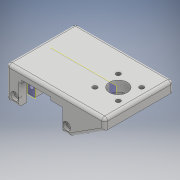
# Autodesk Inventor part: hals
Saved by Autodesk Inventor 2018 (Build 220112000, 112)
## iProperties
Created: 2018-05-22
Part Number: hals
Material: Generic
Document SubType Name: Modeling
Designer: bitbots
Density: 1 g/cm^3
Appearance: Default
Author: bitbots
Autodesk Inventor part; units mm, degrees
ref_plane "YZ Plane" through (0, 0, 0) normal (1, 0, 0) x (0, 1, 0)
ref_plane "XZ Plane" through (0, 0, 0) normal (0, 1, 0) x (-1, 0, 0)
ref_plane "Work Plane1" through (-55.4637, 0, 0.5) normal (0, 0, 1) x (1, 0, 0)
sketch "Sketch1" plane through (-55.4637, 0, 0.5) normal (0, 0, 1) x (1, 0, 0)
  line L0 (-54.3758, 35) -> (-49.4887, 35) projected
  line L1 (-32.4387, 6) -> (-27.5516, 6) projected
  line L2 (-32.4387, 35) -> (-27.5516, 35) projected
  line L3 (-27.5516, 35) -> (-23.5516, 35)
  line L4 (-23.5516, 35) -> (-23.5516, 32.5)
  line L5 (-23.5516, 32.5) -> (-79.5516, 32.5)
  line L6 (-79.5516, 32.5) -> (-79.5516, 8.5)
  line L7 (-79.5516, 8.5) -> (-23.5516, 8.5)
  line L8 (-23.5516, 8.5) -> (-23.5516, 32.5)
  line L9 (-23.5516, 8.5) -> (-22.5516, 8.5)
  line L10 (-22.5516, 8.5) -> (-22.5516, 32.5)
  line L11 (-22.5516, 32.5) -> (-23.5516, 32.5)
  line L12 (-23.5516, 32.5) -> (-23.5516, 8.5)
  point P0 (55.4637, 0)
  dimension "d0" = 4
  dimension "d1" = 2.5
  dimension "d2" = 56
  dimension "d3" = 24
  dimension "d39" = 1
  constraints: 20 end point, 4 parallel, 3 horizontal, 2 perpendicular, 1 vertical
  measures "d0" distance of L2.end L3.end
  measures "d1" distance of L3.end L4.end
  measures "d2" distance of L7.end L6.end
  measures "d3" distance of L6.end L5.end
  measures "d39" distance of L11.end L10.end
extrude "Extrusion1" add sketch "Sketch1" along normal blind 7
ref_plane "Work Plane2" through (-135.0152, 20.5, 7.5) normal (0, 1, 0) x (1, 0, 0)
sketch "Sketch8" plane through (-55.4637, 0, 0.5) normal (0, 0, -1) x (-1, 0, 0)
  circle A0 centre (36.4516, 20.5) radius 5 construction
  circle A1 centre (28.6734, 28.2782) radius 1.025 construction
  circle A2 centre (28.6734, 28.2782) radius 1.5
  circle A3 centre (36.4516, 20.5) radius 6
  circle A4 centre (28.6734, 12.7218) radius 1.5
  circle A5 centre (44.2297, 12.7218) radius 1.5
  circle A6 centre (44.2297, 28.2782) radius 1.5
  point P0 (-55.4637, 0)
  dimension "d40" = 3
  dimension "d41" = 12
  dimension "d44" = 360
  constraints: 5 centre point, 2 coincident, 9 other
  measures "d40" diameter of A2
  measures "d41" diameter of A3
extrude "Extrusion8" cut sketch "Sketch8" against normal through all
sketch "Sketch12" plane through (-55.4637, 0, 0.5) normal (0, 0, -1) x (-1, 0, 0)
  circle A0 centre (44.2297, 28.2782) radius 1.5 construction
  circle A1 centre (28.6734, 12.7218) radius 1.5 construction
  circle A2 centre (28.6734, 28.2782) radius 1.5 construction
  circle A3 centre (44.2297, 12.7218) radius 1.5 construction
  circle A4 centre (36.4516, 20.5) radius 6 construction
  line L0 (79.5516, 8.5) -> (22.5516, 8.5) construction
  line L1 (79.5516, 32.5) -> (79.5516, 8.5) construction
  line L2 (22.5516, 32.5) -> (79.5516, 32.5) construction
  line L3 (22.5516, 8.5) -> (22.5516, 32.5) construction
  circle A5 centre (44.2297, 12.7218) radius 2.75
  circle A6 centre (44.2297, 28.2782) radius 2.75
  circle A7 centre (28.6734, 28.2782) radius 2.75
  circle A8 centre (28.6734, 12.7218) radius 2.75
  point P0 (-55.4637, 0)
  dimension "d66" = 5.5
  dimension "d69" = 360
  constraints: 4 centre point, 1 coincident, 9 other
  measures "d66" diameter of A5
extrude "Extrusion12" cut sketch "Sketch12" against normal blind 3
sketch "Sketch13" plane through (-135.0152, 32.5, 0.5) normal (0, 1, 0) x (1, 0, 0)
  line L0 (57, 0) -> (0, 0) projected
  line L1 (0, 0) -> (0, -7) projected
  line L2 (57, -7) -> (0, -7) projected
  line L3 (57, 0) -> (57, -7) projected
  point P0 (135.0152, 0.5)
extrude "Extrusion13" add sketch "Sketch13" along normal blind 5.5
mirror "Mirror2" about plane through (-135.0152, 20.5, 7.5) normal (0, 1, 0) of "Extrusion13"
sketch "Sketch15" plane through (-135.0152, 38, 0.5) normal (0, 1, 0) x (1, 0, 0)
  line L0 (57, 0) -> (0, 0) construction
  line L1 (0, 0) -> (0, -7) construction
  line L2 (0, -7) -> (57, -7) construction
  line L3 (57, -7) -> (57, 0) construction
  circle A0 centre (-2.819, 9.5) radius 1.35 construction
  circle A1 centre (31.781, 9.5) radius 1.35 construction
  circle A2 centre (-2.819, 9.5) radius 1.5
  circle A3 centre (31.781, 9.5) radius 1.5
  line L4 (0, -3.5) -> (-5, -3.5)
  line L5 (-2.819, 9.5) -> (-2.819, 14.5) construction
  line L6 (-2.819, 9.5) -> (-0.219, 9.5)
  line L7 (-0.219, 9.5) -> (-0.219, 14.5)
  line L8 (-0.219, 14.5) -> (-2.819, 14.5)
  line L9 (-5, -3.5) -> (-5, 14.5)
  line L10 (-5, 14.5) -> (-2.819, 14.5)
  line L11 (31.781, 9.5) -> (29.181, 9.5)
  line L12 (29.181, 9.5) -> (29.181, 14.5)
  line L13 (29.181, 14.5) -> (34.181, 14.5)
  line L14 (-0.219, 9.5) -> (-0.219, -3.5)
  line L15 (29.181, 9.5) -> (29.181, 0)
  line L16 (34.181, 14.5) -> (34.181, 0)
  line L17 (32.5718, 0) -> (38.0718, 0) projected
  line L18 (-5, -3.5) -> (0, -3.5)
  line L19 (0, -3.5) -> (0, -7)
  line L20 (0, -7) -> (-5, -7)
  line L21 (-5, -7) -> (-5, -3.5)
  line L22 (34.181, 0) -> (0, 0)
  line L23 (0, 0) -> (0, -7)
  line L24 (0, -7) -> (34.181, -7)
  line L25 (34.181, -7) -> (34.181, 0)
  line L26 (29.181, 0) -> (34.181, 0)
  line L27 (0, 0) -> (-0.219, 0)
  line L28 (-0.219, 0) -> (-0.219, -3.5)
  line L29 (-0.219, -3.5) -> (0, -3.5)
  line L30 (0, -3.5) -> (0, 0)
  line L31 (34.181, 14.5) -> (57, 0)
  line L32 (57, -7) -> (57, 0) projected
  line L33 (57, 0) -> (57, -7)
  line L34 (36.8218, -7) -> (33.8218, -7) projected
  line L35 (57, -7) -> (33.8218, -7)
  line L36 (34.181, 14.5) -> (34.181, -7)
  line L37 (34.181, -7) -> (57, -7)
  point P0 (135.0152, 0.5)
  dimension "d75" = 3
  dimension "d76" = 3
  dimension "d77" = 5
  dimension "d78" = 5
  dimension "d79" = 2.6
  dimension "d80" = 2.6
  dimension "d81" = 5
  dimension "d82" = 5
  constraints: 62 end point, 10 perpendicular, 8 horizontal, 7 parallel, 4 point on line, 3 collinear, 2 centre point, 2 coincident, 2 vertical, 1 midpoint
  measures "d75" diameter of A2
  measures "d76" diameter of A3
  measures "d77" distance of L4.start L4.end
  measures "d78" distance of L5.start L5.end
  measures "d79" distance of L5.start L6.end
  measures "d80" distance of L11.start L11.end
  measures "d81" distance of L11.end L12.end
  measures "d82" distance of L12.end L13.end
extrude "Extrusion14" add sketch "Sketch15" along normal blind 2
mirror "Mirror3" about plane through (-135.0152, 20.5, 7.5) normal (0, 1, 0) of "Extrusion14"
sketch "Sketch16" plane through (-140.0152, 3, 7.5) normal (0, 1, 0) x (1, 0, 0)
  line L0 (5, 7) -> (5, 0) construction
  line L1 (5, 7) -> (4.781, 7) construction
  line L2 (4.781, 7) -> (4.781, 21.5) construction
  line L3 (4.781, 21.5) -> (0, 21.5) construction
  line L4 (0, 21.5) -> (0, 0) construction
  line L5 (0, 0) -> (5, 0) construction
  circle A0 centre (2.181, 16.5) radius 1.5 construction
  line L6 (0, 21.5) -> (0, 0) construction
  line L7 (0, 0) -> (5, 0) construction
  line L8 (5, 0) -> (4.781, 7) construction
  line L9 (5, 7) -> (5, 0) projected
  line L10 (0, 0) -> (5, 0)
  line L11 (5, 7) -> (4.781, 7) projected
  line L12 (5, 7) -> (4.781, 7)
  line L13 (4.781, 7) -> (0, 11.781)
  line L14 (0, 0) -> (62, 0) projected
  line L15 (0, 11.781) -> (0, 0)
  point P0 (140.0152, 7.5)
  point P1 (39.2, 0)
  dimension "d85" = 135
  constraints: 12 end point, 2 horizontal, 2 perpendicular, 1 point on line
  measures "d85" angle of L12 L13
extrude "Extrusion15" add sketch "Sketch16" along normal up to next
ref_plane "Work Plane3" through (-140.0152, 8.5, -14) normal (0, 1, 0) x (1, 0, 0)
sketch "Sketch17" plane through (-140.0152, 8.5, -14) normal (0, 1, 0) x (1, 0, 0)
  circle A0 centre (2.181, -5) radius 1.5 projected
  circle A1 centre (36.781, -5) radius 1.5 projected
  line L0 (0, -21.5) -> (62, -21.5) construction
  line L1 (62, -21.5) -> (62, -14.5) construction
  line L2 (62, -14.5) -> (39.181, 0) construction
  line L3 (39.181, 0) -> (34.181, 0) construction
  line L4 (34.181, 0) -> (34.181, -14.5) construction
  line L5 (34.181, -14.5) -> (4.781, -14.5) construction
  line L6 (4.781, -14.5) -> (4.781, 0) construction
  line L7 (4.781, 0) -> (0, 0) construction
  line L8 (0, 0) -> (0, -21.5) construction
  line L9 (4.781, -14.5) -> (4.781, 0) projected
  line L10 (0, 0) -> (4.781, 0)
  line L11 (4.781, 0) -> (4.781, -14.5)
  line L12 (4.781, -14.5) -> (0, -14.5)
  line L13 (0, -14.5) -> (0, 0)
  line L14 (41.8218, -21.5) -> (38.8218, -21.5) projected
  line L15 (34.181, 0) -> (40.3218, 0)
  line L16 (40.3218, 0) -> (40.3218, -21.5)
  line L17 (40.3218, -21.5) -> (34.181, -21.5)
  line L18 (34.181, -21.5) -> (34.181, 0)
  point P0 (140.0152, -14)
  constraints: 16 end point, 4 parallel, 2 horizontal, 2 perpendicular, 1 midpoint
extrude "Extrusion16" add sketch "Sketch17" along normal blind 24 contours L12 L13 L10 L9
sketch "Sketch18" plane through (-135.0152, 40, 0.5) normal (0, 1, 0) x (1, 0, 0)
  circle A0 centre (-2.819, 9.5) radius 1.5 projected
  circle A1 centre (31.781, 9.5) radius 1.5 projected
  line L0 (-5, -7) -> (57, -7) projected
  line L1 (57, -7) -> (57, 0) projected
  line L2 (57, 0) -> (34.181, 14.5) projected
  line L3 (34.181, 14.5) -> (29.181, 14.5) projected
  line L4 (29.181, 14.5) -> (29.181, 0) projected
  line L5 (29.181, 0) -> (-0.219, 0) projected
  line L6 (-0.219, 0) -> (-0.219, 14.5) projected
  line L7 (-0.219, 14.5) -> (-5, 14.5) projected
  line L8 (-5, 14.5) -> (-5, -7) projected
  point P0 (135.0152, 0.5)
extrude "Extrusion17" add sketch "Sketch18" along normal blind 1.5
mirror "Mirror4" about plane through (-135.0152, 20.5, 7.5) normal (0, 1, 0) of "Extrusion17"
sketch "Sketch19" plane through (-140.0152, 3, -14) normal (-1, 0, 0) x (0, 0, 1)
  line L0 (6.5, 5.5) -> (6.5, 29.5) projected
  line L1 (9.719, 0) -> (9.719, 5.5) projected
  line L2 (0, 0) -> (9.719, 0) projected
  line L3 (0, 0) -> (0, -3.5) projected
  line L4 (0, -3.5) -> (21.5, -3.5) projected
  line L5 (21.5, -3.5) -> (21.5, 38.5) projected
  line L6 (0, 38.5) -> (21.5, 38.5) projected
  line L7 (0, 35) -> (0, 38.5) projected
  line L8 (0, 35) -> (9.719, 35) projected
  line L9 (9.719, 29.5) -> (9.719, 35) projected
  line L10 (0, 29.5) -> (9.719, 29.5) projected
  line L11 (0, 5.5) -> (0, 29.5) projected
  line L12 (0, 5.5) -> (9.719, 5.5) projected
  point P0 (14, -3)
extrude "Extrusion18" add sketch "Sketch19" along normal blind 1.5
sketch "Sketch20" plane through (-141.5152, 3, -14) normal (-1, 0, 0) x (0, 0, 1)
  line L0 (9.719, 5.5) -> (9.719, 0) projected
  line L1 (9.719, 0) -> (0, 0) projected
  line L2 (0, 0) -> (0, -3.5) projected
  line L3 (0, -3.5) -> (21.5, -3.5) projected
  line L4 (21.5, -3.5) -> (21.5, 38.5) projected
  line L5 (21.5, 38.5) -> (0, 38.5) projected
  line L6 (0, 38.5) -> (0, 35) projected
  line L7 (0, 35) -> (9.719, 35) projected
  line L8 (9.719, 35) -> (9.719, 29.5) projected
  line L9 (9.719, 29.5) -> (0, 29.5) projected
  line L10 (0, 29.5) -> (0, 5.5) projected
  line L11 (0, 5.5) -> (9.719, 5.5) projected
  line L12 (0, 0) -> (0, -3.5) projected
  line L13 (0, 0) -> (9.719, 0)
  line L14 (9.719, 0) -> (9.719, 5.5)
  line L15 (9.719, 5.5) -> (0, 5.5)
  line L16 (0, 5.5) -> (0, 0)
  line L17 (14.5, 35) -> (0, 35) projected
  line L18 (9.719, 29.5) -> (0, 29.5)
  line L19 (0, 29.5) -> (0, 35)
  line L20 (0, 35) -> (9.719, 35)
  line L21 (9.719, 35) -> (9.719, 29.5)
  point P0 (14, -3)
  constraints: 16 end point, 4 parallel, 2 horizontal, 2 perpendicular
extrude "Extrusion19" add sketch "Sketch20" along normal blind 2
sketch "Sketch21" plane through (-55.4637, 0, 0.5) normal (0, 0, -1) x (-1, 0, 0)
  circle A0 centre (36.4516, 20.5) radius 6 construction
  circle A1 centre (28.6734, 12.7218) radius 2.75 construction
  circle A2 centre (44.2297, 28.2782) radius 2.75 construction
  circle A3 centre (44.2297, 12.7218) radius 2.75 construction
  circle A4 centre (28.6734, 28.2782) radius 2.75 construction
  line L0 (79.7706, 3) -> (79.7706, 8.5) construction
  line L1 (79.7706, 8.5) -> (79.7706, 32.5) construction
  line L2 (79.7706, 32.5) -> (79.7706, 38) construction
  line L3 (79.7706, 38) -> (79.7706, 41.5) construction
  line L4 (50.3706, 41.5) -> (79.7706, 41.5) construction
  line L5 (50.3706, 38) -> (50.3706, 41.5) construction
  line L6 (22.5516, 38) -> (50.3706, 38) construction
  line L7 (22.5516, 38) -> (22.5516, 3) construction
  line L8 (22.5516, 3) -> (50.3706, 3) construction
  line L9 (50.3706, 3) -> (50.3706, -0.5) construction
  line L10 (50.3706, -0.5) -> (79.7706, -0.5) construction
  line L11 (79.7706, 3) -> (79.7706, -0.5) construction
  line L12 (50.5706, 35.5) -> (50.5706, 5.5) construction
  line L13 (50.5706, 33) -> (46.6536, 33) construction
  line L14 (45.6336, 8) -> (49.1995, 8) construction
  line L15 (45.6336, 8) -> (49.1995, 8) construction
  line L16 (50.5706, 33) -> (49.5706, 33)
  line L17 (49.5706, 33) -> (49.5706, 32)
  line L18 (49.5706, 32) -> (50.5706, 32)
  line L19 (50.5706, 32) -> (50.5706, 33)
  line L20 (50.5706, 8) -> (49.5706, 8)
  line L21 (49.5706, 8) -> (49.5706, 9)
  line L22 (49.5706, 9) -> (50.5706, 9)
  line L23 (50.5706, 9) -> (50.5706, 8)
  line L24 (49.5706, 32) -> (41.4797, 32)
  line L25 (41.4797, 32) -> (41.4797, 9)
  line L26 (41.4797, 9) -> (49.5706, 9)
  line L27 (49.5706, 9) -> (49.5706, 32)
  line L28 (44.9706, 37.5) -> (44.9706, 35)
  line L29 (45.6336, 8) -> (45.6336, 6)
  line L30 (41.4797, 32) -> (43.9797, 32)
  line L31 (43.9797, 32) -> (43.9797, 37.5)
  line L32 (43.9797, 37.5) -> (41.4797, 37.5)
  line L33 (41.4797, 37.5) -> (41.4797, 32)
  line L34 (22.5516, 3) -> (50.3706, 3)
  line L35 (41.4797, 9) -> (43.9797, 9)
  line L36 (43.9797, 9) -> (43.9797, 3)
  line L37 (43.9797, 3) -> (41.4797, 3)
  line L38 (41.4797, 3) -> (41.4797, 9)
  line L39 (22.5516, 38) -> (50.3706, 38)
  line L40 (43.9797, 37.5) -> (41.4797, 37.5)
  line L41 (41.4797, 37.5) -> (41.4797, 38)
  line L42 (41.4797, 38) -> (43.9797, 38)
  line L43 (43.9797, 38) -> (43.9797, 37.5)
  point P0 (-55.4637, 0)
extrude "Extrusion20" add sketch "Sketch21" along normal blind 14.5 contours L27 L26 L25 L24 | L24 L33 L32 L31 | L32 L41 L39 L43 | L36 L34 L38 L26
sketch "Sketch22" plane through (-55.4637, 0, 0.5) normal (0, 0, -1) x (-1, 0, 0)
  circle A0 centre (44.2297, 12.7218) radius 2.75 projected
  circle A1 centre (44.2297, 28.2782) radius 2.75 projected
  point P0 (-55.4637, 0)
extrude "Extrusion21" cut sketch "Sketch22" along normal blind 15
sketch "Sketch23" plane through (-135.0152, 41.5, 0.5) normal (0, 1, 0) x (1, 0, 0)
  circle A0 centre (31.781, 9.5) radius 1.5 projected
  point P0 (135.0152, 0.5)
extrude "Extrusion22" cut sketch "Sketch23" against normal through all
sketch "Sketch24" plane through (-135.0152, 41.5, 0.5) normal (0, 1, 0) x (1, 0, 0)
  circle A0 centre (31.781, 9.5) radius 1.5 projected
  circle A1 centre (-2.819, 9.5) radius 1.5 projected
  line L0 (57, -7) -> (-8.5, -7) projected
  line L1 (57, -7) -> (57, 0) projected
  line L2 (57, 0) -> (34.181, 14.5) projected
  line L3 (34.181, 14.5) -> (29.181, 14.5) projected
  line L4 (29.181, 14.5) -> (29.181, 0) projected
  line L5 (29.181, 0) -> (-0.219, 0) projected
  line L6 (-0.219, 0) -> (-0.219, 14.5) projected
  line L7 (-0.219, 14.5) -> (-8.5, 14.5) projected
  line L8 (-8.5, -7) -> (-8.5, 14.5) projected
  circle A2 centre (-2.819, 9.5) radius 2.6
  circle A3 centre (31.781, 9.5) radius 2.6
  point P0 (135.0152, 0.5)
  dimension "d111" = 5.2
  dimension "d112" = 5.2
  constraints: 2 centre point, 2 coincident
  measures "d111" diameter of A2
  measures "d112" diameter of A3
extrude "Extrusion23" add sketch "Sketch24" along normal blind 2 contours L0 L8 L7 L6 L5 L4 L3 L2 L1
mirror "Mirror5" about plane through (-135.0152, 20.5, 7.5) normal (0, 1, 0) of "Extrusion23"
chamfer "Chamfer2" distance 2.4 angle 45 2 edges at (-98.1934, 38, -14) (-98.1934, 3, -14)
sketch "Sketch25" plane through (-55.4637, 0, 0.5) normal (0, 0, -1) x (-1, 0, 0)
  line L0 (77.7706, -2.5) -> (58.3706, -2.5)
  line L1 (58.3706, -2.5) -> (58.3706, 0)
  line L2 (58.3706, 0) -> (77.7706, 0)
  line L3 (77.7706, 0) -> (77.7706, -2.5)
  line L4 (77.7706, 43.5) -> (77.7706, 38) projected
  line L5 (77.7706, 43.5) -> (58.3706, 43.5)
  line L6 (58.3706, 43.5) -> (58.3706, 41)
  line L7 (58.3706, 41) -> (77.7706, 41)
  line L8 (77.7706, 41) -> (77.7706, 43.5)
  point P0 (-55.4637, 0)
  point P1 (52.3706, -2.5)
  dimension "d120" = 19.4
  dimension "d121" = 2.5
  dimension "d122" = 19.4
  dimension "d123" = 2.5
  constraints: 16 end point, 4 parallel, 2 horizontal, 2 perpendicular
  measures "d120" distance of L1.end L2.end
  measures "d121" distance of L0.end L1.end
  measures "d122" distance of L7.end L6.end
  measures "d123" distance of L6.end L5.end
extrude "Extrusion24" cut sketch "Sketch25" against normal blind 2
fillet "Fillet1" radius 2 17 edges at (-89.4248, 43.5, -6.75) (-100.8343, 40.75, -14) (-100.8343, 0.25, -14) (-89.4248, -2.5, -6.75) (-143.5152, 20.5, 7.5) (-110.7652, 43.5, 7.5) (-143.5152, 43.5, -3.25) (-143.5152, 20.5, -14) (-143.5152, -2.5, -3.25) (-110.7652, -2.5, 7.5) (-78.0152, 20.5, 7.5) (-78.0152, 43.5, 4) (-78.0152, -2.5, 4) (-139.3748, 43.5, -14) (-139.3748, -2.5, -14) (-103.3343, 43.5, -14) (-103.3343, -2.5, -14)
body "Solid1"
